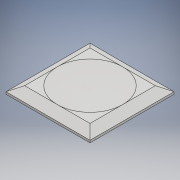
# Autodesk Inventor part: 障害物、窪地
Saved by Autodesk Inventor 2017 (Build 210142000, 142)
## iProperties
Part Number: 障害物、窪地
Material: 一般
Document SubType Name: Modeling
Designer: 雪村
Density: 1 g/cm^3
Appearance: 既定
Mass: 5766.95 g
Surface Area: 4401.15 cm^2
Volume: 5766.95 cm^3
Author: 雪村
Autodesk Inventor part; units mm, degrees
ref_plane "YZ Plane" through (0, 0, 0) normal (1, 0, 0) x (0, 1, 0)
ref_plane "XZ Plane" through (0, 0, 0) normal (0, 1, 0) x (-1, 0, 0)
sketch "スケッチ1" plane through (0, 0, 0) normal (0, 0, 1) x (1, 0, 0)
  line L0 (-225, 225) -> (225, 225)
  line L1 (225, 225) -> (225, -225)
  line L2 (225, -225) -> (-225, -225)
  line L3 (-225, -225) -> (-225, 225)
  point P0 (0, 0)
  point P1 (0, 0)
  dimension "d0" = 450
  constraints: 8 end point, 1 coincident, 1 horizontal, 9 other
  measures "d0" distance of L0.start L0.end
extrude "押し出し1" add sketch "スケッチ1" along normal blind 12
sketch "スケッチ2" plane through (0, 0, 12) normal (0, 0, 1) x (1, 0, 0)
  line L0 (225, 225) -> (-225, 225) projected
  line L1 (-225, 225) -> (-225, -225) projected
  line L2 (-225, -225) -> (225, -225) projected
  line L3 (225, -225) -> (225, 225) projected
  point P0 (0, 0)
extrude "押し出し2" add sketch "スケッチ2" along normal blind 28
chamfer "面取り1" distance 50 distance2 28 1 edges at (0, 225, 40) measured on face at (-75, -75, 40)
chamfer "面取り2" distance 50 distance2 28 1 edges at (0, -225, 40) measured on face at (-75, 41.6667, 40)
chamfer "面取り3" distance 50 distance2 28 1 edges at (-225, 0, 40) measured on face at (-75, 58.3333, 40)
chamfer "面取り4" distance 50 distance2 28 1 edges at (225, 0, 40) measured on face at (-41.6667, -58.3333, 40)
ref_plane "作業平面2" through (-225, 0, 0) normal (0, -1, 0) x (1, 0, 0)
ref_plane "作業平面1" through (-225, 225, 0) normal (0, -1, 0) x (1, 0, 0)
sketch "スケッチ6" plane through (-225, 0, 0) normal (0, -1, 0) x (1, 0, 0)
  line L0 (225, 0) -> (225, 15)
  line L1 (50, 40) -> (0, 12) projected
  arc A0 (50, 40) -> (225, 15) centre (235.7026, 714.9182) ccw
  line L2 (50, 40) -> (225, 40.2475)
  line L3 (225, 40.2475) -> (225, 15)
  dimension "d18" = 15
  dimension "d19" = 700
  dimension "d20" = 175.0002
  constraints: 6 end point, 2 point on circle, 2 vertical, 1 centre point
  measures "d18" distance of L0.start L0.end
  measures "d19" radius of A0
  measures "d20" distance of L1.start L2.end
revolve "回転1" cut sketch "スケッチ6" angle 360 about axis through (0, 0, 40.2475) along (0, 0, -1)
sketch "スケッチ7" plane through (0, 0, 0) normal (0, 0, -1) x (-1, 0, 0)
  circle A0 centre (0, 0) radius 0.005
  dimension "d22" = 0.01
  constraints: 1 centre point, 1 coincident
  measures "d22" diameter of A0
extrude "押し出し3" cut sketch "スケッチ7" against normal through all
